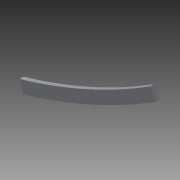
# Autodesk Inventor part: nd-7
Saved by Autodesk Inventor 2015 (Build 190159000, 159)
## iProperties
Created: 2014-07-02
Part Number: nd-7
Material: Generic
Document SubType Name: Modeling
Designer: peter
Density: 1 g/cm^3
Appearance: Default
Author: peter
Autodesk Inventor part; units mm, degrees
ref_plane "YZ Plane" through (0, 0, 0) normal (1, 0, 0) x (0, 1, 0)
ref_plane "XZ Plane" through (0, 0, 0) normal (0, 1, 0) x (-1, 0, 0)
ref_plane "XY Plane" through (0, 0, 0) normal (0, 0, 1) x (1, 0, 0)
sketch "Sketch1" plane through (0, 0, 0) normal (0, 0, 1) x (1, 0, 0)
  line L0 (623.87, 336.0812) -> (654.4461, 287.7984)
  arc A0 (161.0048, 46.9938) -> (654.4461, 287.7984) centre (-677.3108, 2390.7821) ccw
  arc A1 (16.0036, 0.0852) -> (161.0048, 46.9938) centre (-677.3108, 2390.7821) ccw
  line L1 (16.0036, 0.0852) -> (0.0857, 54.9736)
  arc A2 (0.0857, 54.9736) -> (141.7866, 100.8156) centre (-677.3108, 2390.7821) ccw
  arc A3 (141.7866, 100.8156) -> (623.87, 336.0812) centre (-677.3108, 2390.7821) ccw
  constraints: 8 point on circle, 4 centre point, 4 end point
extrude "Extrusion1" add sketch "Sketch1" along normal blind 19.05
body "Solid1"
